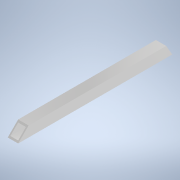
# Autodesk Inventor part: aluminumBallHandlerBackLeg
Saved by Autodesk Inventor 2020.2 (Build 242310000, 310)
## iProperties
Created: 2020-01-16
Part Number: aluminumBallHandlerBackLeg
Material: Aluminum 6061-AHC
Document SubType Name: Modeling
Designer: robst
Density: 2.7 g/cm^3
Appearance: Aluminum - Dark
Author: robst
Autodesk Inventor part; units mm, degrees
ref_plane "YZ Plane" through (0, 0, 0) normal (1, 0, 0) x (0, 1, 0)
ref_plane "XZ Plane" through (0, 0, 0) normal (0, 1, 0) x (-1, 0, 0)
ref_plane "XY Plane" through (0, 0, 0) normal (0, 0, 1) x (1, 0, 0)
sketch "Sketch2" plane through (0, 0, 0) normal (0, 0, 1) x (1, 0, 0)
  line L0 (-12.7, -12.7) -> (12.7, -12.7)
  line L1 (12.7, -12.7) -> (12.7, 12.7)
  line L2 (12.7, 12.7) -> (-12.7, 12.7)
  line L3 (-12.7, 12.7) -> (-12.7, -12.7)
  line L4 (-12.7, -12.7) -> (12.7, 12.7) construction
  line L5 (12.7, -12.7) -> (-12.7, 12.7) construction
  line L6 (-9.525, -9.525) -> (9.525, -9.525)
  line L7 (9.525, -9.525) -> (9.525, 9.525)
  line L8 (9.525, 9.525) -> (-9.525, 9.525)
  line L9 (-9.525, 9.525) -> (-9.525, -9.525)
  line L10 (-9.525, -9.525) -> (9.525, 9.525) construction
  line L11 (9.525, -9.525) -> (-9.525, 9.525) construction
  point P0 (0, 0)
  dimension "d0" = 25.4
  dimension "d1" = 25.4
  dimension "d2" = 3.175
  dimension "d3" = 3.175
  constraints: 24 end point, 5 parallel, 4 midpoint, 2 perpendicular, 1 horizontal
  measures "d0" distance of L0.start L0.end
  measures "d1" distance of L1.end L0.end
  measures "d2" distance between parallel lines of L6 L0
  measures "d3" distance between parallel lines of L9 L3
extrude "Extrusion1" add sketch "Sketch2" along normal mid plane 346.6084
sketch "Sketch5" plane through (12.7, -12.7, -173.3042) normal (1, 0, 0) x (0, 0, -1)
  line L0 (0, 0) -> (-14.6647, 25.4)
  line L1 (0, 25.4) -> (-346.6084, 25.4) projected
  line L2 (-346.6084, 0) -> (0, 0) projected
  line L3 (-14.6647, 25.4) -> (0, 25.4)
  line L4 (0, 0) -> (0, 25.4) projected
  line L5 (0, 25.4) -> (0, 0)
  point P0 (-173.3042, 12.7)
  point P1 (-557.2214, 25.4)
  point P2 (-601.2155, 0)
  dimension "d10" = 60
  constraints: 6 end point, 2 collinear, 1 point on line
  measures "d10" angle of L0 L2
extrude "Extrusion3" cut sketch "Sketch5" against normal through all
sketch "Sketch6" plane through (12.7, -12.7, 173.3042) normal (1, 0, 0) x (0, 0, -1)
  line L0 (0, 0) -> (0, 25.4) projected
  line L1 (0, 0) -> (25.4, 25.4)
  line L2 (331.9437, 25.4) -> (0, 25.4) projected
  line L3 (0, 0) -> (346.6084, 0) projected
  line L4 (25.4, 25.4) -> (0, 25.4)
  line L5 (0, 25.4) -> (0, 0)
  point P0 (173.3042, 12.7)
  dimension "d13" = 45
  constraints: 6 end point, 1 collinear, 1 perpendicular, 1 point on line
  measures "d13" angle of L1 L3
extrude "Extrusion4" cut sketch "Sketch6" against normal through all
body "Solid1"
